Autodesk Inventor part; units mm, degrees
(part 3 of 3)
  line L1853 (6.5731, 14.3966) -> (6.6336, 14.3361)
  line L1854 (6.6336, 14.3361) -> (6.6557, 14.2534)
  line L1855 (6.6557, 14.2534) -> (6.6191, 14.1749)
  line L1856 (6.6191, 14.1749) -> (6.5731, 14.1102)
  line L1857 (6.4904, 14.0881) -> (6.4077, 14.1102)
  line L1858 (6.4077, 14.1102) -> (6.3472, 14.1708)
  line L1859 (6.3472, 14.1708) -> (6.3168, 14.2617)
  line L1860 (5.3008, 14.0051) -> (5.3291, 14.0816)
  line L1861 (5.3896, 14.1421) -> (5.4723, 14.1642)
  line L1862 (5.4723, 14.1642) -> (5.555, 14.1421)
  line L1863 (5.555, 14.1421) -> (5.6155, 14.0816)
  line L1864 (5.6155, 14.0816) -> (5.6376, 13.9989)
  line L1865 (5.6155, 13.9162) -> (5.555, 13.8557)
  line L1866 (5.555, 13.8557) -> (5.4723, 13.8336)
  line L1867 (5.4723, 13.8336) -> (5.3896, 13.8557)
  line L1868 (-5.8382, 16.4996) -> (-5.8151, 16.4178)
  line L1869 (-5.8151, 16.4178) -> (-5.8382, 16.3342)
  line L1870 (-5.8382, 16.3342) -> (-5.8987, 16.2737)
  line L1871 (-5.8987, 16.2737) -> (-5.9813, 16.2516)
  line L1872 (-5.9813, 16.2516) -> (-6.064, 16.2737)
  line L1873 (-6.064, 16.2737) -> (-6.1117, 16.3308)
  line L1874 (-6.1117, 16.3308) -> (-6.1467, 16.4169)
  line L1875 (-6.1467, 15.1443) -> (-6.1245, 15.2269)
  line L1876 (-6.1245, 15.2269) -> (-6.064, 15.2875)
  line L1877 (-6.064, 15.2875) -> (-5.9813, 15.3096)
  line L1878 (-5.9813, 15.3096) -> (-5.8987, 15.2875)
  line L1879 (-5.8987, 15.2875) -> (-5.8382, 15.2269)
  line L1880 (-5.8382, 15.2269) -> (-5.8116, 15.1487)
  line L1881 (-5.8116, 15.1487) -> (-5.8382, 15.0616)
  line L1882 (-5.8382, 15.0616) -> (-5.8987, 15.0011)
  line L1883 (-5.8987, 15.0011) -> (-5.9813, 14.9789)
  line L1884 (-5.9813, 14.9789) -> (-6.064, 15.0011)
  line L1885 (-6.064, 15.0011) -> (-6.1128, 15.0609)
  line L1886 (-6.1128, 15.0609) -> (-6.1467, 15.1443)
  line L1887 (-4.365, 15.1443) -> (-4.3429, 15.2269)
  line L1888 (-4.3429, 15.2269) -> (-4.2823, 15.2875)
  line L1889 (-4.2823, 15.2875) -> (-4.1997, 15.3096)
  line L1890 (-4.1997, 15.3096) -> (-4.117, 15.2875)
  line L1891 (-4.117, 15.2875) -> (-4.0565, 15.2269)
  line L1892 (-4.0565, 15.2269) -> (-4.0348, 15.1438)
  line L1893 (-4.0348, 15.1438) -> (-4.0565, 15.0616)
  line L1894 (-4.0565, 15.0616) -> (-4.117, 15.0011)
  line L1895 (-4.117, 15.0011) -> (-4.1997, 14.9789)
  line L1896 (-4.1997, 14.9789) -> (-4.2823, 15.0011)
  line L1897 (-4.2823, 15.0011) -> (-4.3409, 15.0611)
  line L1898 (-4.3409, 15.0611) -> (-4.365, 15.1443)
  line L1899 (-12.4718, 11.2883) -> (-12.5466, 11.3126)
  line L1900 (-12.5466, 11.3126) -> (-12.6149, 11.371)
  line L1901 (-12.6149, 11.371) -> (-12.6371, 11.4536)
  line L1902 (-15.5641, 10.5628) -> (-15.542, 10.6455)
  line L1903 (-15.542, 10.6455) -> (-15.4815, 10.706)
  line L1904 (-15.4815, 10.706) -> (-15.3988, 10.7282)
  line L1905 (-15.3988, 10.7282) -> (-15.3161, 10.706)
  line L1906 (-15.3161, 10.706) -> (-15.2536, 10.6529)
  line L1907 (-15.2536, 10.6529) -> (-15.2335, 10.5628)
  line L1908 (-15.2335, 10.5628) -> (-15.2556, 10.4801)
  line L1909 (-15.2556, 10.4801) -> (-15.3161, 10.4196)
  line L1910 (-15.3161, 10.4196) -> (-15.3988, 10.3975)
  line L1911 (-15.4815, 10.4196) -> (-15.542, 10.4801)
  line L1912 (-15.542, 10.4801) -> (-15.5641, 10.5628)
  line L1913 (-2.3288, 16.9259) -> (-2.3067, 17.0086)
  line L1914 (-2.3067, 17.0086) -> (-2.2461, 17.0691)
  line L1915 (-2.2461, 17.0691) -> (-2.1635, 17.0913)
  line L1916 (-2.1635, 17.0913) -> (-2.0808, 17.0691)
  line L1917 (-2.0808, 17.0691) -> (-2.0203, 17.0086)
  line L1918 (-2.0203, 17.0086) -> (-2.0092, 16.9149)
  line L1919 (-2.0092, 16.9149) -> (-2.0203, 16.8433)
  line L1920 (-2.0203, 16.8433) -> (-2.0808, 16.7828)
  line L1921 (-2.0808, 16.7828) -> (-2.1635, 16.7606)
  line L1922 (-2.1635, 16.7606) -> (-2.2461, 16.7828)
  line L1923 (-2.2461, 16.7828) -> (-2.3067, 16.8433)
  line L1924 (-13.6552, 10.4355) -> (-13.633, 10.5182)
  line L1925 (-13.633, 10.5182) -> (-13.5725, 10.5787)
  line L1926 (-13.5725, 10.5787) -> (-13.4899, 10.6009)
  line L1927 (-13.4899, 10.6009) -> (-13.4072, 10.5787)
  line L1928 (-13.4072, 10.5787) -> (-13.3452, 10.5237)
  line L1929 (-13.3452, 10.5237) -> (-13.3245, 10.4355)
  line L1930 (-13.3245, 10.4355) -> (-13.3467, 10.3529)
  line L1931 (-13.3467, 10.3529) -> (-13.4072, 10.2924)
  line L1932 (-13.4072, 10.2924) -> (-13.4899, 10.2702)
  line L1933 (-13.4899, 10.2702) -> (-13.5581, 10.2962)
  line L1934 (-13.5581, 10.2962) -> (-13.633, 10.3529)
  line L1935 (-13.633, 10.3529) -> (-13.6552, 10.4355)
  line L1936 (-14.2915, 3.6906) -> (-14.2694, 3.7733)
  line L1937 (-14.2694, 3.7733) -> (-14.2088, 3.8338)
  line L1938 (-14.2088, 3.8338) -> (-14.1262, 3.856)
  line L1939 (-14.1262, 3.856) -> (-14.0484, 3.8347)
  line L1940 (-14.0484, 3.8347) -> (-13.983, 3.7733)
  line L1941 (-13.983, 3.7733) -> (-13.9608, 3.6906)
  line L1942 (-13.9608, 3.6906) -> (-13.983, 3.6079)
  line L1943 (-13.983, 3.6079) -> (-14.0435, 3.5474)
  line L1944 (-14.0435, 3.5474) -> (-14.1306, 3.5279)
  line L1945 (-14.1306, 3.5279) -> (-14.2088, 3.5474)
  line L1946 (-14.2088, 3.5474) -> (-14.2694, 3.6079)
  line L1947 (-14.2694, 3.6079) -> (-14.2915, 3.6906)
  line L1948 (-17.6003, -0.7636) -> (-17.5782, -0.6809)
  line L1949 (-17.5782, -0.6809) -> (-17.5177, -0.6204)
  line L1950 (-17.5177, -0.6204) -> (-17.435, -0.5982)
  line L1951 (-17.3523, -0.6204) -> (-17.2918, -0.6809)
  line L1952 (-17.2918, -0.6809) -> (-17.2697, -0.7636)
  line L1953 (-17.2697, -0.7636) -> (-17.2918, -0.8462)
  line L1954 (-17.2918, -0.8462) -> (-17.3557, -0.9193)
  line L1955 (-17.3557, -0.9193) -> (-17.435, -0.9289)
  line L1956 (-17.435, -0.9289) -> (-17.5177, -0.9068)
  line L1957 (-17.5177, -0.9068) -> (-17.5782, -0.8462)
  line L1958 (-17.5782, -0.8462) -> (-17.6003, -0.7636)
  line L1959 (-16.3277, -0.6363) -> (-16.3056, -0.5536)
  line L1960 (-16.3056, -0.5536) -> (-16.245, -0.4931)
  line L1961 (-16.245, -0.4931) -> (-16.1556, -0.4904)
  line L1962 (-16.1556, -0.4904) -> (-16.0797, -0.4931)
  line L1963 (-16.0797, -0.4931) -> (-16.0192, -0.5536)
  line L1964 (-16.0192, -0.5536) -> (-15.997, -0.6363)
  line L1965 (-15.997, -0.6363) -> (-16.0192, -0.719)
  line L1966 (-16.0192, -0.719) -> (-16.0837, -0.7945)
  line L1967 (-16.0837, -0.7945) -> (-16.1624, -0.8017)
  line L1968 (-16.1624, -0.8017) -> (-16.245, -0.7795)
  line L1969 (-16.245, -0.7795) -> (-16.3056, -0.719)
  line L1970 (-16.3056, -0.719) -> (-16.3277, -0.6363)
  line L1971 (-15.1823, -5.7268) -> (-15.1602, -5.6442)
  line L1972 (-15.1602, -5.6442) -> (-15.0997, -5.5836)
  line L1973 (-15.0997, -5.5836) -> (-15.0211, -5.5574)
  line L1974 (-15.0211, -5.5574) -> (-14.9343, -5.5836)
  line L1975 (-14.9343, -5.5836) -> (-14.8738, -5.6442)
  line L1976 (-14.8738, -5.6442) -> (-14.8517, -5.7268)
  line L1977 (-14.8517, -5.7268) -> (-14.8738, -5.8095)
  line L1978 (-14.8738, -5.8095) -> (-14.9343, -5.8597)
  line L1979 (-14.9343, -5.8597) -> (-15.017, -5.8922)
  line L1980 (-15.017, -5.8922) -> (-15.0997, -5.87)
  line L1981 (-15.0997, -5.87) -> (-15.1602, -5.8095)
  line L1982 (-15.1602, -5.8095) -> (-15.1823, -5.7268)
  line L1983 (-13.7825, -5.9813) -> (-13.7603, -5.8987)
  line L1984 (-13.7603, -5.8987) -> (-13.6998, -5.8382)
  line L1985 (-13.6998, -5.8382) -> (-13.6257, -5.8074)
  line L1986 (-13.6257, -5.8074) -> (-13.5344, -5.8382)
  line L1987 (-13.5344, -5.8382) -> (-13.4739, -5.8987)
  line L1988 (-13.4739, -5.8987) -> (-13.4518, -5.9813)
  line L1989 (-13.4518, -5.9813) -> (-13.4739, -6.064)
  line L1990 (-13.4739, -6.064) -> (-13.5421, -6.1128)
  line L1991 (-13.5421, -6.1128) -> (-13.6171, -6.1467)
  line L1992 (-13.6171, -6.1467) -> (-13.6998, -6.1245)
  line L1993 (-13.6998, -6.1245) -> (-13.7603, -6.064)
  line L1994 (-13.7603, -6.064) -> (-13.7825, -5.9813)
  line L1995 (-14.2915, -8.0176) -> (-14.2694, -7.9349)
  line L1996 (-14.2694, -7.9349) -> (-14.2088, -7.8744)
  line L1997 (-14.2088, -7.8744) -> (-14.139, -7.8394)
  line L1998 (-14.139, -7.8394) -> (-14.0435, -7.8744)
  line L1999 (-14.0435, -7.8744) -> (-13.983, -7.9349)
  line L2000 (-13.983, -7.9349) -> (-13.9608, -8.0176)
  line L2001 (-13.9608, -8.0176) -> (-13.978, -8.119)
  line L2002 (-13.978, -8.119) -> (-14.0435, -8.1607)
  line L2003 (-14.0435, -8.1607) -> (-14.1262, -8.1829)
  line L2004 (-14.1262, -8.1829) -> (-14.2088, -8.1607)
  line L2005 (-14.2088, -8.1607) -> (-14.2694, -8.1002)
  line L2006 (-14.2694, -8.1002) -> (-14.2915, -8.0176)
  line L2007 (-12.5098, -12.3445) -> (-12.4877, -12.2618)
  line L2008 (-12.4877, -12.2618) -> (-12.4212, -12.2029)
  line L2009 (-12.4212, -12.2029) -> (-12.3445, -12.1791)
  line L2010 (-12.3445, -12.1791) -> (-12.2618, -12.2013)
  line L2011 (-12.2618, -12.2013) -> (-12.2013, -12.2618)
  line L2012 (-12.2013, -12.2618) -> (-12.1791, -12.3445)
  line L2013 (-12.1791, -12.3445) -> (-12.2029, -12.4212)
  line L2014 (-12.2029, -12.4212) -> (-12.2618, -12.4877)
  line L2015 (-12.2618, -12.4877) -> (-12.3445, -12.5098)
  line L2016 (-12.3445, -12.5098) -> (-12.4272, -12.4877)
  line L2017 (-12.4272, -12.4877) -> (-12.4877, -12.4272)
  line L2018 (-12.4877, -12.4272) -> (-12.5098, -12.3445)
  line L2019 (-8.8192, -13.8716) -> (-8.7971, -13.789)
  line L2020 (-8.7971, -13.789) -> (-8.7517, -13.7244)
  line L2021 (-8.7517, -13.7244) -> (-8.6539, -13.7063)
  line L2022 (-8.6539, -13.7063) -> (-8.5712, -13.7285)
  line L2023 (-8.5712, -13.7285) -> (-8.5107, -13.789)
  line L2024 (-8.5107, -13.789) -> (-8.4885, -13.8716)
  line L2025 (-8.5107, -13.9543) -> (-8.5712, -14.0148)
  line L2026 (-8.5712, -14.0148) -> (-8.6539, -14.037)
  line L2027 (-8.6539, -14.037) -> (-8.7365, -14.0148)
  line L2028 (-8.7365, -14.0148) -> (-8.7971, -13.9543)
  line L2029 (-8.7971, -13.9543) -> (-8.8192, -13.8716)
  line L2030 (0.7435, -15.3962) -> (0.7476, -15.3161)
  line L2031 (0.7476, -15.3161) -> (0.8082, -15.2556)
  line L2032 (0.8082, -15.2556) -> (0.8908, -15.2335)
  line L2033 (0.8908, -15.2335) -> (0.9735, -15.2556)
  line L2034 (0.9735, -15.2556) -> (1.0487, -15.3201)
  line L2035 (1.0487, -15.3201) -> (1.0562, -15.3988)
  line L2036 (1.0562, -15.3988) -> (1.034, -15.4815)
  line L2037 (1.034, -15.4815) -> (0.9735, -15.542)
  line L2038 (0.9735, -15.542) -> (0.8908, -15.5641)
  line L2039 (0.8908, -15.5641) -> (0.8082, -15.542)
  line L2040 (0.8082, -15.542) -> (0.7476, -15.4815)
  line L2041 (0.7476, -15.4815) -> (0.7435, -15.3962)
  line L2042 (13.3245, -13.4899) -> (13.3467, -13.4072)
  line L2043 (13.3467, -13.4072) -> (13.4072, -13.3467)
  line L2044 (13.4072, -13.3467) -> (13.4899, -13.3245)
  line L2045 (13.4899, -13.3245) -> (13.5623, -13.3494)
  line L2046 (13.5623, -13.3494) -> (13.633, -13.4072)
  line L2047 (13.633, -13.4072) -> (13.6552, -13.4899)
  line L2048 (13.6552, -13.4899) -> (13.633, -13.5725)
  line L2049 (13.633, -13.5725) -> (13.5725, -13.633)
  line L2050 (13.3467, -13.5725) -> (13.3245, -13.4899)
  line L2051 (13.07, 10.5628) -> (13.0909, 10.6499)
  line L2052 (13.0909, 10.6499) -> (13.1527, 10.706)
  line L2053 (13.1527, 10.706) -> (13.2353, 10.7282)
  line L2054 (13.2353, 10.7282) -> (13.318, 10.706)
  line L2055 (13.318, 10.706) -> (13.3785, 10.6455)
  line L2056 (13.3785, 10.6455) -> (13.4007, 10.5628)
  line L2057 (13.4007, 10.5628) -> (13.3785, 10.4801)
  line L2058 (13.3785, 10.4801) -> (13.305, 10.4231)
  line L2059 (13.305, 10.4231) -> (13.2353, 10.3975)
  line L2060 (13.2353, 10.3975) -> (13.1527, 10.4196)
  line L2061 (13.1527, 10.4196) -> (13.0921, 10.4801)
  line L2062 (13.0921, 10.4801) -> (13.07, 10.5628)
  line L2063 (11.161, 12.8535) -> (11.1832, 12.9362)
  line L2064 (11.2437, 12.9967) -> (11.3264, 13.0189)
  line L2065 (11.4696, 12.9362) -> (11.4917, 12.8535)
  line L2066 (-17.6003, 4.0724) -> (-17.5782, 4.1551)
  line L2067 (-17.5782, 4.1551) -> (-17.5177, 4.2156)
  line L2068 (-17.5177, 4.2156) -> (-17.435, 4.2377)
  line L2069 (-17.435, 4.2377) -> (-17.3511, 4.2112)
  line L2070 (-17.3511, 4.2112) -> (-17.2918, 4.1551)
  line L2071 (-17.2918, 4.1551) -> (-17.2697, 4.0724)
  line L2072 (-17.2697, 4.0724) -> (-17.2918, 3.9897)
  line L2073 (-17.2918, 3.9897) -> (-17.3523, 3.9292)
  line L2074 (-17.3523, 3.9292) -> (-17.4278, 3.9142)
  line L2075 (-17.4278, 3.9142) -> (-17.5177, 3.9292)
  line L2076 (-17.5177, 3.9292) -> (-17.5782, 3.9897)
  line L2077 (-17.5782, 3.9897) -> (-17.6003, 4.0724)
  line L2078 (-17.6003, 2.5453) -> (-17.5782, 2.6279)
  line L2079 (-17.5782, 2.6279) -> (-17.5177, 2.6884)
  line L2080 (-17.5177, 2.6884) -> (-17.435, 2.7106)
  line L2081 (-17.435, 2.7106) -> (-17.3532, 2.6918)
  line L2082 (-17.3532, 2.6918) -> (-17.2918, 2.6279)
  line L2083 (-17.2918, 2.6279) -> (-17.2697, 2.5453)
  line L2084 (-17.2697, 2.5453) -> (-17.2918, 2.4626)
  line L2085 (-17.2918, 2.4626) -> (-17.3523, 2.4021)
  line L2086 (-17.3523, 2.4021) -> (-17.4236, 2.3913)
  line L2087 (-17.4236, 2.3913) -> (-17.5177, 2.4021)
  line L2088 (-17.5177, 2.4021) -> (-17.5782, 2.4626)
  line L2089 (-1.4445, 3.7065) -> (-1.384, 3.646)
  line L2090 (-1.3618, 3.5634) -> (-1.384, 3.4807)
  line L2091 (-1.4445, 3.4202) -> (-1.5272, 3.398)
  line L2092 (-1.5272, 3.398) -> (-1.6098, 3.4202)
  line L2093 (-1.6098, 3.4202) -> (-1.6703, 3.4807)
  line L2094 (-1.6703, 3.4807) -> (-1.6925, 3.5634)
  line L2095 (-5.2337, -0.0827) -> (-5.2559, 0)
  line L2096 (1.2567, 12.2999) -> (1.3172, 12.3604)
  line L2097 (1.3172, 12.3604) -> (1.3999, 12.3826)
  line L2098 (1.3999, 12.3826) -> (1.4826, 12.3604)
  line L2099 (1.4826, 12.3604) -> (1.5431, 12.2999)
  line L2100 (1.5431, 12.2999) -> (1.5652, 12.2172)
  line L2101 (1.5652, 12.2172) -> (1.5566, 12.1499)
  line L2102 (1.5566, 12.1499) -> (1.4826, 12.074)
  line L2103 (1.4826, 12.074) -> (1.3999, 12.0519)
  line L2104 (1.3999, 12.0519) -> (1.3172, 12.074)
  line L2105 (1.3172, 12.074) -> (1.2567, 12.1346)
  line L2106 (1.2567, 12.1346) -> (1.2345, 12.2172)
  line L2107 (-3.4742, 12.7263) -> (-3.452, 12.8089)
  line L2108 (-3.452, 12.8089) -> (-3.3915, 12.8695)
  line L2109 (-3.3915, 12.8695) -> (-3.3088, 12.8916)
  line L2110 (-3.3088, 12.8916) -> (-3.2262, 12.8695)
  line L2111 (-3.2262, 12.8695) -> (-3.1656, 12.8089)
  line L2112 (-3.1656, 12.8089) -> (-3.1482, 12.7384)
  line L2113 (-3.1482, 12.7384) -> (-3.1656, 12.6436)
  line L2114 (-3.1656, 12.6436) -> (-3.2262, 12.5831)
  line L2115 (-3.2262, 12.5831) -> (-3.3088, 12.5609)
  line L2116 (-3.3088, 12.5609) -> (-3.3915, 12.5831)
  line L2117 (-3.3915, 12.5831) -> (-3.455, 12.6562)
  line L2118 (-3.455, 12.6562) -> (-3.4742, 12.7263)
  line L2119 (-2.5833, 11.8354) -> (-2.5612, 11.9181)
  line L2120 (-2.5007, 11.9786) -> (-2.418, 12.0008)
  line L2121 (-2.418, 12.0008) -> (-2.3353, 11.9786)
  line L2122 (-2.3353, 11.9786) -> (-2.2748, 11.9181)
  line L2123 (-2.2748, 11.9181) -> (-2.2623, 11.8525)
  line L2124 (-2.2623, 11.8525) -> (-2.2748, 11.7528)
  line L2125 (-2.2748, 11.7528) -> (-2.3353, 11.6922)
  line L2126 (-2.3353, 11.6922) -> (-2.418, 11.6701)
  line L2127 (-2.418, 11.6701) -> (-2.5007, 11.6922)
  line L2128 (-2.5007, 11.6922) -> (-2.5691, 11.7703)
  line L2129 (-2.5691, 11.7703) -> (-2.5833, 11.8354)
  line L2130 (-1.3107, 13.1081) -> (-1.2886, 13.1907)
  line L2131 (-1.2886, 13.1907) -> (-1.228, 13.2513)
  line L2132 (-1.228, 13.2513) -> (-1.1454, 13.2734)
  line L2133 (-1.1454, 13.2734) -> (-1.0627, 13.2513)
  line L2134 (-1.0627, 13.2513) -> (-1.0022, 13.1907)
  line L2135 (-1.0022, 13.1907) -> (-0.9967, 13.1181)
  line L2136 (-0.9967, 13.1181) -> (-1.0022, 13.0254)
  line L2137 (-1.0022, 13.0254) -> (-1.0627, 12.9649)
  line L2138 (-1.0627, 12.9649) -> (-1.1454, 12.9427)
  line L2139 (-1.1454, 12.9427) -> (-1.228, 12.9649)
  line L2140 (-1.228, 12.9649) -> (-1.3035, 13.0359)
  line L2141 (-1.3035, 13.0359) -> (-1.3107, 13.1081)
  line L2142 (4.1607, 12.9915) -> (4.1837, 13.0635)
  line L2143 (4.1837, 13.0635) -> (4.2443, 13.124)
  line L2144 (4.2443, 13.124) -> (4.3269, 13.1461)
  line L2145 (4.3269, 13.1461) -> (4.4096, 13.124)
  line L2146 (4.4096, 13.124) -> (4.4701, 13.0635)
  line L2147 (4.4701, 13.0635) -> (4.4923, 12.9808)
  line L2148 (4.4923, 12.9808) -> (4.4675, 12.9093)
  line L2149 (4.4675, 12.9093) -> (4.4096, 12.8376)
  line L2150 (4.4096, 12.8376) -> (4.3269, 12.8155)
  line L2151 (4.3269, 12.8155) -> (4.2443, 12.8376)
  line L2152 (4.2443, 12.8376) -> (4.1837, 12.8981)
  line L2153 (4.1837, 12.8981) -> (4.1607, 12.9915)
  line L2154 (1.2567, 8.6093) -> (1.3172, 8.6698)
  line L2155 (1.3172, 8.6698) -> (1.3999, 8.6919)
  line L2156 (1.3999, 8.6919) -> (1.4826, 8.6698)
  line L2157 (1.4826, 8.6698) -> (1.5431, 8.6093)
  line L2158 (1.5431, 8.4439) -> (1.4826, 8.3834)
  line L2159 (1.3999, 8.3613) -> (1.3172, 8.3834)
  line L2160 (1.3172, 8.3834) -> (1.2567, 8.4439)
  line L2161 (1.2567, 8.4439) -> (1.2345, 8.5266)
  line L2162 (15.0253, 7.0804) -> (14.9343, 7.1108)
  line L2163 (14.8517, 4.7087) -> (14.8738, 4.7914)
  line L2164 (14.8738, 4.7914) -> (14.9343, 4.8472)
  line L2165 (14.9343, 4.8472) -> (15.017, 4.8741)
  line L2166 (15.017, 4.8741) -> (15.0997, 4.8519)
  line L2167 (15.0997, 4.8519) -> (15.1602, 4.7914)
  line L2168 (15.1602, 4.7914) -> (15.1823, 4.7087)
  line L2169 (15.1823, 4.7087) -> (15.1602, 4.6261)
  line L2170 (15.1602, 4.6261) -> (15.0997, 4.5655)
  line L2171 (15.0997, 4.5655) -> (15.0183, 4.5421)
  line L2172 (15.0183, 4.5421) -> (14.9343, 4.5655)
  line L2173 (14.9343, 4.5655) -> (14.8738, 4.6261)
  line L2174 (14.8738, 4.6261) -> (14.8517, 4.7087)
  line L2175 (15.542, -0.719) -> (15.4815, -0.7795)
  line L2176 (-13.5279, 2.1635) -> (-13.5058, 2.2461)
  line L2177 (-13.3626, 2.3288) -> (-13.289, 2.316)
  line L2178 (-13.289, 2.316) -> (-13.2194, 2.2461)
  line L2179 (-13.2194, 2.2461) -> (-13.1972, 2.1635)
  line L2180 (-13.1972, 2.1635) -> (-13.2194, 2.0808)
  line L2181 (-13.2194, 2.0808) -> (-13.2799, 2.0203)
  line L2182 (-13.2799, 2.0203) -> (-13.3712, 2.0092)
  line L2183 (-13.3712, 2.0092) -> (-13.4453, 2.0203)
  line L2184 (-13.4453, 2.0203) -> (-13.5058, 2.0808)
  line L2185 (-13.5058, 2.0808) -> (-13.5279, 2.1635)
  line L2186 (-14.7784, 2.5007) -> (-14.7179, 2.5612)
  line L2187 (-14.7179, 2.5612) -> (-14.6352, 2.5833)
  line L2188 (-14.6352, 2.5833) -> (-14.5547, 2.5691)
  line L2189 (-14.5547, 2.5691) -> (-14.492, 2.5007)
  line L2190 (-14.492, 2.5007) -> (-14.4699, 2.418)
  line L2191 (-14.4699, 2.418) -> (-14.492, 2.3353)
  line L2192 (-14.492, 2.3353) -> (-14.5525, 2.2748)
  line L2193 (-14.5525, 2.2748) -> (-14.6368, 2.2623)
  line L2194 (-14.6368, 2.2623) -> (-14.7179, 2.2748)
  line L2195 (-14.7179, 2.2748) -> (-14.7784, 2.3353)
  line L2196 (-14.7784, 2.3353) -> (-14.8006, 2.418)
  line L2197 (2.5293, 3.7733) -> (2.5898, 3.8338)
  line L2198 (2.8379, 3.6906) -> (2.8157, 3.6079)
  line L2199 (2.6725, 3.5253) -> (2.5898, 3.5474)
  line L2200 (2.5898, 3.5474) -> (2.5293, 3.6079)
  line L2201 (2.5293, 3.6079) -> (2.5072, 3.6906)
  line L2202 (0.7255, 3.6906) -> (0.7476, 3.7733)
  line L2203 (0.8908, 3.856) -> (0.9735, 3.8338)
  line L2204 (1.034, 3.7733) -> (1.0562, 3.6906)
  line L2205 (1.034, 3.6079) -> (0.9735, 3.5474)
  line L2206 (0.9735, 3.5474) -> (0.8908, 3.5253)
  line L2207 (0.8908, 3.5253) -> (0.8082, 3.5474)
  line L2208 (0.8082, 3.5474) -> (0.7476, 3.6079)
  line L2209 (0.7476, 3.6079) -> (0.7255, 3.6906)
  line L2210 (-11.2372, -2.1635) -> (-11.215, -2.0808)
  line L2211 (-11.215, -2.0808) -> (-11.1545, -2.0203)
  line L2212 (-11.0719, -1.9981) -> (-10.9892, -2.0203)
  line L2213 (-10.9892, -2.0203) -> (-10.9287, -2.0808)
  line L2214 (-10.9287, -2.0808) -> (-10.9065, -2.1635)
  line L2215 (-11.215, -2.2461) -> (-11.2372, -2.1635)
  line L2216 (-17.0913, 7.1267) -> (-17.0691, 7.2094)
  line L2217 (-17.0691, 7.2094) -> (-17.0086, 7.2699)
  line L2218 (-17.0086, 7.2699) -> (-16.9259, 7.2921)
  line L2219 (-16.9259, 7.2921) -> (-16.8381, 7.2505)
  line L2220 (-16.8381, 7.2505) -> (-16.7828, 7.2094)
  line L2221 (-16.7828, 7.2094) -> (-16.7606, 7.1267)
  line L2222 (-16.7606, 7.1267) -> (-16.7828, 7.044)
  line L2223 (-16.7828, 7.044) -> (-16.8433, 6.9835)
  line L2224 (-16.8433, 6.9835) -> (-16.9286, 6.9587)
  line L2225 (-16.9286, 6.9587) -> (-17.0086, 6.9835)
  line L2226 (-17.0086, 6.9835) -> (-17.0691, 7.044)
  line L2227 (-17.0691, 7.044) -> (-17.0913, 7.1267)
  line L2228 (-8.0176, 7.763) -> (-7.9835, 7.8903)
  line L2229 (-7.9835, 7.8903) -> (-7.8903, 7.9835)
  line L2230 (-7.8903, 7.9835) -> (-7.763, 8.0176)
  line L2231 (-7.763, 8.0176) -> (-7.6358, 7.9835)
  line L2232 (-7.5426, 7.8903) -> (-7.5085, 7.763)
  line L2233 (-7.5085, 7.763) -> (-7.5426, 7.6358)
  line L2234 (-7.5426, 7.6358) -> (-7.6358, 7.5426)
  line L2235 (-7.6358, 7.5426) -> (-7.763, 7.5085)
  line L2236 (-7.763, 7.5085) -> (-7.8903, 7.5426)
  line L2237 (-7.9835, 7.6358) -> (-8.0176, 7.763)
  line L2238 (7.5085, 7.763) -> (7.5426, 7.8903)
  line L2239 (7.6358, 7.9835) -> (7.763, 8.0176)
  line L2240 (7.763, 8.0176) -> (7.8903, 7.9835)
  line L2241 (7.8903, 7.9835) -> (7.9835, 7.8903)
  line L2242 (7.9835, 7.8903) -> (8.0176, 7.763)
  line L2243 (8.0176, 7.763) -> (7.9835, 7.6358)
  line L2244 (7.8903, 7.5426) -> (7.763, 7.5085)
  line L2245 (7.763, 7.5085) -> (7.6358, 7.5426)
  line L2246 (7.6358, 7.5426) -> (7.5426, 7.6358)
  line L2247 (7.5426, 7.6358) -> (7.5085, 7.763)
  line L2248 (-7.763, -7.5085) -> (-7.6358, -7.5426)
  line L2249 (-7.8903, -7.9835) -> (-7.9835, -7.8903)
  line L2250 (-7.9835, -7.8903) -> (-8.0176, -7.763)
  line L2251 (7.5085, -7.763) -> (7.5426, -7.6358)
  line L2252 (7.9835, -7.6358) -> (8.0176, -7.763)
  line L2253 (8.0176, -7.763) -> (7.9835, -7.8903)
  line L2254 (7.9835, -7.8903) -> (7.8903, -7.9835)
  line L2255 (7.8903, -7.9835) -> (7.763, -8.0176)
  line L2256 (7.763, -8.0176) -> (7.6358, -7.9835)
  line L2257 (1.3035, 5.6953) -> (1.3107, 5.7268)
  line L2258 (1.5566, 8.4796) -> (1.5652, 8.5266)
  line L2259 (-1.3763, 3.6259) -> (-1.384, 3.646)
  line L2260 (1.0504, 3.6703) -> (1.0562, 3.6906)
  line L2261 (2.8002, 3.5881) -> (2.8157, 3.6079)
  line L2262 (-0.7255, 17.435) -> (-0.7435, 17.4212)
  line L2263 (13.3245, 16.6714) -> (13.3384, 16.7234)
  line L2264 (13.3384, 16.7234) -> (13.3467, 16.7541)
  line L2265 (14.7716, 16.1624) -> (15.0609, 16.444)
  line L2266 (15.0609, 16.444) -> (15.1443, 16.535)
  line L2267 (15.1443, -11.4156) -> (15.2033, -11.4349)
  line L2268 (15.2033, -11.4349) -> (15.2269, -11.4377)
  line L2269 (7.8903, -7.5426) -> (7.9395, -7.5937)
  line L2270 (7.9395, -7.5937) -> (7.9835, -7.6358)
  line L2271 (0.7476, 17.3523) -> (0.7364, 17.3944)
  line L2272 (0.7364, 17.3944) -> (0.7255, 17.435)
  line L2273 (2.8157, 3.7733) -> (2.8002, 3.7525)
  line L2274 (2.8002, 3.7525) -> (2.8379, 3.6906)
  line L2275 (-3.7525, -2.0092) -> (-3.6906, -1.9981)
  line L2276 (-16.535, -15.1443) -> (-16.444, -15.0609)
  line L2277 (-16.444, -15.0609) -> (-16.1624, -14.7716)
  line L2278 (8.9675, 13.7444) -> (8.9277, 13.7046)
  line L2279 (8.9277, 13.7046) -> (8.7811, 13.5581)
  line L2280 (18.0967, -14.055) -> (17.997, -13.9776)
  line L2281 (17.997, -13.9776) -> (17.7589, -13.846)
  line L2282 (16.535, 15.1443) -> (16.444, 15.0609)
  line L2283 (16.444, 15.0609) -> (16.1624, 14.7716)
  line L2284 (14.1005, -17.7589) -> (14.2307, -17.997)
  line L2285 (14.2307, -17.997) -> (14.3095, -18.0967)
  line L2286 (15.3988, -16.535) -> (15.314, -16.444)
  line L2287 (15.314, -16.444) -> (15.0261, -16.1624)
  line L2288 (16.4169, -14.7716) -> (16.6971, -15.0609)
  line L2289 (16.6971, -15.0609) -> (16.7895, -15.1443)
  line L2290 (-3.6906, -2.3288) -> (-3.7525, -2.294)
  line L2291 (-3.7525, -2.294) -> (-3.7733, -2.3067)
  line L2292 (8.077, 18.3515) -> (7.9701, 18.1449)
  line L2293 (2.5898, 3.8338) -> (2.6578, 3.8347)
  line L2294 (2.6578, 3.8347) -> (2.6725, 3.856)
  line L2295 (15.9905, 12.9649) -> (15.9637, 12.9577)
  line L2296 (15.9637, 12.9577) -> (15.9078, 12.9427)
  line L2297 (-8.1378, 15.0609) -> (-8.1607, 15.0616)
  line L2298 (-7.5912, 16.2737) -> (-7.6316, 16.3265)
  line L2299 (-7.6316, 16.3265) -> (-7.6517, 16.3342)
  line L2300 (-10.4196, 15.4815) -> (-10.4224, 15.4564)
  line L2301 (-10.4224, 15.4564) -> (-10.3975, 15.3988)
  line L2302 (-7.5426, -7.8903) -> (-7.5937, -7.9395)
  line L2303 (-7.5937, -7.9395) -> (-7.6358, -7.9835)
  line L2304 (-17.3523, 8.1607) -> (-17.339, 8.1378)
  line L2305 (-17.339, 8.1378) -> (-17.2918, 8.1002)
  line L2306 (-10.9892, -2.3067) -> (-11.0109, -2.316)
  line L2307 (-11.0109, -2.316) -> (-11.0719, -2.3288)
  line L2308 (-5.0905, -0.1653) -> (-5.1447, -0.1424)
  line L2309 (-5.1447, -0.1424) -> (-5.1732, -0.1432)
  line L2310 (-5.1732, 0.1432) -> (-5.1447, 0.1424)
  line L2311 (-5.1447, 0.1424) -> (-5.0905, 0.1653)
  line L2312 (-5.0625, 0.1644) -> (-5.0078, 0.1432)
  line L2313 (-13.1972, -17.435) -> (-13.2099, -17.4822)
  line L2314 (-13.2099, -17.4822) -> (-13.2194, -17.5177)
  line L2315 (-15.6533, -2.0453) -> (-15.5671, -2.0341)
  line L2316 (-15.5671, -2.0341) -> (-15.1443, -1.9089)
  line L2317 (-14.6352, -3.8087) -> (-15.062, -3.9231)
  line L2318 (-15.062, -3.9231) -> (-15.1443, -3.9451)
  line L2319 (13.1763, 15.2715) -> (13.289, 15.3727)
  line L2320 (13.289, 15.3727) -> (13.3626, 15.4579)
  line L2321 (13.982, 14.6865) -> (13.8716, 14.5762)
  line L2322 (8.0176, 16.0351) -> (8.0692, 16.2279)
  line L2323 (8.0692, 16.2279) -> (8.0858, 16.2896)
  line L2324 (8.9675, 15.7806) -> (8.9318, 15.7449)
  line L2325 (8.9318, 15.7449) -> (8.7811, 15.5943)
  line L2326 (-14.3807, 9.3794) -> (-14.4439, 9.4099)
  line L2327 (-14.4439, 9.4099) -> (-14.4634, 9.4015)
  line L2328 (15.0997, 11.4377) -> (15.0767, 11.4349)
  line L2329 (15.0767, 11.4349) -> (15.017, 11.4156)
  line L2330 (15.0997, 9.147) -> (15.0767, 9.1568)
  line L2331 (-4.8268, 16.4169) -> (-4.9359, 16.8327)
  line L2332 (-4.9359, 16.8327) -> (-4.9632, 16.9259)
  line L2333 (9.1788, 17.3523) -> (9.1503, 17.339)
  line L2334 (8.0176, 13.9989) -> (8.0733, 14.207)
  line L2335 (8.0733, 14.207) -> (8.0858, 14.2534)
  line L2336 (8.9037, 17.4814) -> (8.8925, 17.5177)
  line L2337 (-14.7716, -16.1624) -> (-15.0609, -16.444)
  line L2338 (-15.0609, -16.444) -> (-15.1443, -16.535)
  line L2339 (-3.0634, 17.435) -> (-3.0466, 17.339)
  line L2340 (-3.0466, 17.339) -> (-2.927, 16.9259)
  line L2341 (1.0022, 5.8095) -> (1.0568, 5.8377)
  line L2342 (1.0568, 5.8377) -> (1.0627, 5.87)
  line L2343 (1.2886, 5.8095) -> (1.2815, 5.7775)
  line L2344 (1.2815, 5.7775) -> (1.3107, 5.7268)
  line L2345 (1.3035, 5.6953) -> (1.2886, 5.6442)
  line L2346 (11.688, 17.4814) -> (11.6922, 17.5177)
  line L2347 (-8.3547, 17.2918) -> (-8.391, 17.339)
  line L2348 (-8.391, 17.339) -> (-8.4153, 17.3523)
  line L2349 (-17.4212, 0.7435) -> (-17.435, 0.7255)
  line L2350 (-17.3904, -10.4196) -> (-17.3548, -10.4224)
  line L2351 (-17.0086, -11.9468) -> (-16.9751, -11.9412)
  line L2352 (-16.9751, -11.9412) -> (-16.9259, -11.9246)
  line L2353 (-17.2631, -13.4739) -> (-17.2296, -13.4649)
  line L2354 (-17.2296, -13.4649) -> (-17.1805, -13.4518)
  line L2355 (-10.9065, -15.3988) -> (-10.9287, -15.4564)
  line L2356 (-10.9287, -15.4564) -> (-10.9287, -15.4815)
  line L2357 (-10.9287, -17.4814) -> (-10.9287, -17.5177)
  line L2358 (-8.9243, -17.3523) -> (-8.8972, -17.339)
  line L2359 (8.8925, -14.9724) -> (8.9037, -14.9501)
  line L2360 (13.4739, -15.9905) -> (13.467, -15.9645)
  line L2361 (13.467, -15.9645) -> (13.4518, -15.9078)
  line L2362 (15.0011, -17.3904) -> (14.9925, -17.3585)
  line L2363 (14.9925, -17.3585) -> (14.9789, -17.3077)
  line L2364 (17.435, -14.5971) -> (17.4844, -14.6104)
  line L2365 (17.4844, -14.6104) -> (17.5177, -14.6193)
  line L2366 (15.6533, -13.1972) -> (15.7111, -13.2127)
  line L2367 (15.7111, -13.2127) -> (15.736, -13.2194)
  line L2368 (17.435, 0.7255) -> (17.3944, 0.7364)
  line L2369 (17.3944, 0.7364) -> (17.3523, 0.7476)
  line L2370 (17.339, 9.4034) -> (17.3523, 9.4334)
  line L2371 (17.5177, 11.4377) -> (17.4814, 11.4349)
  line L2372 (17.2631, 12.7103) -> (17.2284, 12.701)
  line L2373 (17.2284, 12.701) -> (17.1805, 12.6882)
  line L2374 (13.9608, 17.435) -> (13.9738, 17.4834)
  line L2375 (13.9738, 17.4834) -> (13.983, 17.5177)
  line L2376 (12.6882, 17.435) -> (12.7006, 17.4814)
  line L2377 (12.7006, 17.4814) -> (12.7103, 17.5177)
  line L2378 (10.6755, 17.4814) -> (10.6741, 17.5177)
  line L2379 (16.245, 11.6922) -> (16.2158, 11.688)
  line L2380 (16.2158, 11.688) -> (16.1624, 11.6701)
  line L2381 (-15.3988, 10.3975) -> (-15.4564, 10.4224)
  line L2382 (-15.4564, 10.4224) -> (-15.4815, 10.4196)
  line L2383 (-17.435, -0.5982) -> (-17.4212, -0.617)
  line L2384 (-8.524, -13.9376) -> (-8.5107, -13.9543)
  line L2385 (-1.6925, 3.5634) -> (-1.6611, 3.6259)
  line L2386 (-1.6611, 3.6259) -> (-1.6703, 3.646)
  line L2387 (-1.5272, 3.7287) -> (-1.5187, 3.7082)
  line L2388 (-1.5187, 3.7082) -> (-1.4445, 3.7065)
  line L2389 (-1.3763, 3.6259) -> (-1.3618, 3.5634)
  line L2390 (1.2345, 12.2172) -> (1.2498, 12.2322)
  line L2391 (1.2498, 12.2322) -> (1.2567, 12.2999)
  line L2392 (-3.856, -2.1635) -> (-3.8347, -2.1516)
  line L2393 (-3.8347, -2.1516) -> (-3.8338, -2.0808)
  line L2394 (1.2345, 8.5266) -> (1.2498, 8.5619)
  line L2395 (1.2498, 8.5619) -> (1.2567, 8.6093)
  line L2396 (1.5431, 8.6093) -> (1.5346, 8.5619)
  line L2397 (1.5346, 8.5619) -> (1.5652, 8.5266)
  line L2398 (1.5566, 8.4796) -> (1.5431, 8.4439)
  line L2399 (2.8002, 3.5881) -> (2.7552, 3.5474)
  line L2400 (0.8082, 3.8338) -> (0.8859, 3.8347)
  line L2401 (0.8859, 3.8347) -> (0.8908, 3.856)
  line L2402 (0.9735, 3.8338) -> (0.9681, 3.8127)
  line L2403 (0.9681, 3.8127) -> (1.034, 3.7733)
  line L2404 (1.0504, 3.6703) -> (1.034, 3.6079)
  line L2405 (-11.1545, -2.0203) -> (-11.0931, -2.0092)
  line L2406 (-11.0931, -2.0092) -> (-11.0719, -1.9981)
  line L2407 (-7.6358, 7.9835) -> (-7.5937, 7.9395)
  line L2408 (-7.5937, 7.9395) -> (-7.5426, 7.8903)
  line L2409 (-7.8903, 7.5426) -> (-7.9395, 7.5937)
  line L2410 (-7.9395, 7.5937) -> (-7.9835, 7.6358)
  line L2411 (7.5426, 7.8903) -> (7.5937, 7.9395)
  line L2412 (7.5937, 7.9395) -> (7.6358, 7.9835)
  line L2413 (7.9835, 7.6358) -> (7.9395, 7.5937)
  line L2414 (7.9395, 7.5937) -> (7.8903, 7.5426)
  line L2415 (-7.9835, -7.6358) -> (-7.9395, -7.5937)
  line L2416 (-7.9395, -7.5937) -> (-7.8903, -7.5426)
  line L2417 (7.6358, -7.9835) -> (7.5937, -7.9395)
  line L2418 (7.5937, -7.9395) -> (7.5426, -7.8903)
  line L2419 (-0.7364, 17.3944) -> (-0.7476, 17.3523)
  line L2420 (-8.1002, 15.0011) -> (-8.1297, 15.0306)
  line L2421 (-17.3523, 0.7476) -> (-17.3944, 0.7364)
  line L2422 (-17.3931, -0.6095) -> (-17.3523, -0.6204)
  line L2423 (-8.4885, -13.8716) -> (-8.4997, -13.9134)
  line L2424 (18.4531, -14.2304) -> (18.4528, -14.5799)
  dimension "d0" = 36.9062
  constraints: 4850 end point
  measures "d0" distance between parallel lines of L251 L470
extrude "Extrusion1" add sketch "PCB" along normal blind 0.6604 contours L0 L225 L276 L231 L233 L295 L298 L304 L303 L281 L279 L252 L255 L253 L326 L329 L332 L333 L334 L335 L337 L339 L2285 L2284 L340 L341 L342 L343 L346 L347 L349 L351 L352 L354 L356 L358 L360 L361 L362 L363 L364 L366 L369 L374 L375 L376 L378 L382 L384 L386 L387 L388 L390 L391 L393 L395 L397 L400 L402 L404 L406 L408 L409 L411 L412 L414 L418 L420 L424 L428 L430 L431 L433 L434 L436 L437 L438 L441 L442 L444 L445 L448 L449 L451 L452 L454 L456 L457 L458 L460 L461 L462 L463 L465 L466 L467 L470 L472 L474 L475 L477 L478 L479 L480 L481 L483 L484 L485 L487 L488 L491 L493 L494 L495 L496 L497 L499 L501 L502 L504 L506 L510 L512 L514 L516 L517 L518 L520 L522 L523 L524 L527 L528 L530 L532 L534 L536 L537 L539 L540 L541 L543 L545 L546 L547 L2292 L548 L551 L552 L554 L556 L559 L560 L561 L562 L563 L564 L565 L568 L570 L571 L572 L573 L575 L576 L577 L578 L579 L580 L581 L582 L584 L251 L261 L264 L248 L284 L293 L222 L292 L250 L223 L288 L289 L294 L299 L291 L273 L260 L275 L263 L268 L271 L306 L308 L2281 L2280 L311 L2424 L318 L320 L323
move or copy body "Move Body1" bodies to move or copy 1 copy no rotation origin (0, 0, 0) rotation axis (0.5773503, 0.5773503, 0.5773503) rotation angle -120
sketch "Sketch3" plane through (-6.6988, 0.6604, 18.4531) normal (0, 1, 0) x (1, 0, 0)
  line L0 (25.1319, 36.8662) -> (25.1319, 0.0158) construction
  line L1 (25.1319, 0.0158) -> (-11.7186, 0.0158) construction
  line L2 (-11.7186, 0.0158) -> (-11.7186, 36.8662) construction
  line L3 (-11.7186, 36.8662) -> (25.1319, 36.8662) construction
  point P0 (6.6988, 18.4531)
  constraints: 2 other
decal "Decal1"
sketch "Sketch4" plane through (-6.6988, 0, 18.4531) normal (0, -1, 0) x (1, 0, 0)
  line L0 (25.0402, 0.0345) -> (25.0402, -36.8159) construction
  line L1 (25.0402, -36.8159) -> (-11.8103, -36.8159) construction
  line L2 (-11.8103, -36.8159) -> (-11.8103, 0.0345) construction
  line L3 (-11.8103, 0.0345) -> (25.0402, 0.0345) construction
  point P0 (6.6988, -18.4531)
  constraints: 2 other
decal "Decal2"
body "Solid1"
